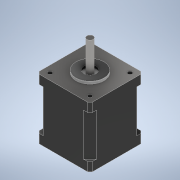
# Autodesk Inventor part: Nema17
Saved by Autodesk Inventor 2021 (Build 250183000, 183)
## iProperties
Created: 2021-04-05
Part Number: Nema17
Material: Gold
Document SubType Name: Modeling
Designer: jorge
Density: 19.3 g/cm^3
Appearance: Glossy - Black
Author: jorge
Autodesk Inventor part; units mm, degrees
ref_plane "YZ Plane" through (0, 0, 0) normal (1, 0, 0) x (0, 1, 0)
ref_plane "XZ Plane" through (0, 0, 0) normal (0, 1, 0) x (-1, 0, 0)
ref_plane "XY Plane" through (0, 0, 0) normal (0, 0, 1) x (1, 0, 0)
sketch "Sketch1" plane through (0, 0, 0) normal (0, 1, 0) x (-1, 0, 0)
  line L0 (0, 0) -> (-42, 0)
  line L1 (-42, 0) -> (-42, -42)
  line L2 (-42, -42) -> (0, -42)
  line L3 (0, -42) -> (0, 0)
  dimension "d0" = 42
  dimension "d1" = 42
  constraints: 8 end point, 2 parallel, 1 horizontal, 1 perpendicular
  measures "d0" distance of L2.end L1.end
  measures "d1" distance of L1.end L0.end
extrude "Extrusion1" add sketch "Sketch1" along normal blind 47.5
chamfer "Chamfer1" distance 5 angle 45 4 edges at (42, 23.75, 0) (0, 23.75, 0) (0, 23.75, -42) (42, 23.75, -42)
sketch "Sketch3" plane through (0, 47.5, 0) normal (0, 1, 0) x (1, 0, 0)
  line L0 (0, 0) -> (42, 0)
  line L1 (42, 0) -> (42, 42)
  line L2 (42, 42) -> (0, 42)
  line L3 (0, 42) -> (0, 0)
  line L4 (37, 42) -> (5, 42) projected
  line L5 (42, 5) -> (42, 37) projected
  constraints: 8 end point, 2 collinear, 2 parallel, 1 horizontal, 1 perpendicular
extrude "Extrusion2" add sketch "Sketch3" against normal blind 7
sketch "Sketch4" plane through (0, 0, 0) normal (0, -1, 0) x (1, 0, 0)
  line L0 (0, 0) -> (42, 0) projected
  line L1 (0, -42) -> (0, 0) projected
  line L2 (42, 0) -> (0, 0)
  line L3 (0, 0) -> (0, -42)
  line L4 (0, -42) -> (42, -42)
  line L5 (42, -42) -> (42, 0)
  constraints: 8 end point, 2 parallel, 1 horizontal, 1 perpendicular
extrude "Extrusion3" add sketch "Sketch4" against normal blind 7
chamfer "Chamfer2" distance 2 angle 45 8 edges at (42, 44, 0) (42, 3.5, 0) (42, 44, -42) (42, 3.5, -42) (0, 3.5, -42) (0, 3.5, 0) (0, 44, 0) (0, 44, -42)
sketch "Sketch5" plane through (0, 0, 0) normal (0, -1, 0) x (1, 0, 0)
  circle A0 centre (21, -21) radius 5
  line L0 (40, -42) -> (2, -42) projected
  line L1 (42, -40) -> (42, -2) projected
  point P0 (0, 0)
  dimension "d14" = 10
  dimension "d15" = 21
  dimension "d16" = 21
  constraints: 1 centre point
  measures "d14" diameter of A0
  measures "d15" distance from line of A0.centre L0
  measures "d16" distance from line of A0.centre L1
extrude "Extrusion4" cut sketch "Sketch5" against normal blind 7
sketch "Sketch6" plane through (0, 47.5, 0) normal (0, 1, 0) x (1, 0, 0)
  circle A0 centre (21, 21) radius 5 projected
  circle A1 centre (21, 21) radius 5
  circle A2 centre (21, 21) radius 11
  point P0 (0, 0)
  dimension "d19" = 10
  dimension "d20" = 22
  constraints: 2 centre point, 2 coincident
  measures "d19" diameter of A1
  measures "d20" diameter of A2
extrude "Extrusion5" add sketch "Sketch6" along normal blind 2
sketch "Sketch7" plane through (0, 47.5, 0) normal (0, 1, 0) x (1, 0, 0)
  circle A0 centre (5.25, 5.25) radius 1.6
  circle A1 centre (5.25, 36.75) radius 1.6
  circle A2 centre (36.75, 36.75) radius 1.6
  circle A3 centre (36.75, 5.25) radius 1.6
  line L0 (2, 0) -> (40, 0) projected
  line L1 (0, 40) -> (0, 2) projected
  point P0 (0, 0)
  dimension "d23" = 3.2
  dimension "d24" = 3.2
  dimension "d25" = 3.2
  dimension "d26" = 3.2
  dimension "d27" = 31.5
  dimension "d28" = 31.5
  dimension "d29" = 31.5
  dimension "d30" = 31.5
  dimension "d31" = 5.25
  dimension "d32" = 5.25
  dimension "d33" = 5.25
  dimension "d34" = 5.25
  constraints: 4 centre point
  measures "d23" diameter of A0
  measures "d24" diameter of A1
  measures "d25" diameter of A2
  measures "d26" diameter of A3
  measures "d27" distance of A1.centre A0.centre
  measures "d28" distance of A2.centre A1.centre
  measures "d29" distance of A3.centre A0.centre
  measures "d30" distance of A2.centre A3.centre
  measures "d31" distance from line of L0 A0.centre
  measures "d32" distance from line of L1 A0.centre
  measures "d33" distance from line of L1 A1.centre
  measures "d34" distance from line of L0 A3.centre
extrude "Extrusion6" cut sketch "Sketch7" against normal blind 10
sketch "Sketch8" plane through (0, 0, 0) normal (0, -1, 0) x (1, 0, 0)
  circle A0 centre (5.25, -36.75) radius 1.6 projected
  circle A1 centre (5.25, -36.75) radius 1.6
  circle A2 centre (5.25, -5.25) radius 1.6 projected
  circle A3 centre (5.25, -5.25) radius 1.6
  circle A4 centre (36.75, -36.75) radius 1.6 projected
  circle A5 centre (36.75, -36.75) radius 1.6
  circle A6 centre (36.75, -5.25) radius 1.6 projected
  circle A7 centre (36.75, -5.25) radius 1.6
  point P0 (0, 0)
  dimension "d37" = 3.2
  dimension "d38" = 3.2
  dimension "d39" = 3.2
  dimension "d40" = 3.2
  constraints: 4 centre point, 4 coincident
  measures "d37" diameter of A1
  measures "d38" diameter of A3
  measures "d39" diameter of A5
  measures "d40" diameter of A7
extrude "Extrusion7" cut sketch "Sketch8" against normal blind 2
sketch "Sketch9" plane through (21, 47.5, -21) normal (0, 1, 0) x (1, 0, 0)
  circle A0 centre (0, 0) radius 2.5
  line L0 (-21, 19) -> (-21, -19) projected
  line L1 (-19, -21) -> (19, -21) projected
  point P0 (-21, -21)
  dimension "d43" = 5
  dimension "d44" = 21
  dimension "d45" = 21
  constraints: 1 centre point
  measures "d43" diameter of A0
  measures "d44" distance from line of A0.centre L0
  measures "d45" distance from line of L1 A0.centre
extrude "Extrusion8" add sketch "Sketch9" along normal blind 24
body "Solid1"
